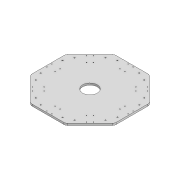
# Autodesk Inventor part: Base
Saved by Autodesk Inventor 2020 (Build 240168000, 168)
## iProperties
Created: 2022-03-01
Part Number: Base
Material: Generic
Document SubType Name: Modeling
Designer: ferrerx
Density: 1 g/cm^3
Appearance: Default
Author: ferrerx
Autodesk Inventor part; units mm, degrees
ref_plane "YZ Plane" through (0, 0, 0) normal (1, 0, 0) x (0, 1, 0)
ref_plane "XZ Plane" through (0, 0, 0) normal (0, 1, 0) x (-1, 0, 0)
ref_plane "XY Plane" through (0, 0, 0) normal (0, 0, 1) x (1, 0, 0)
sketch "Sketch1" plane through (0, 0, 0) normal (0, 1, 0) x (-1, 0, 0)
  circle A0 centre (0, 0) radius 20
  circle A1 centre (0, 0) radius 92.5 construction
  line L0 (115, -37.3658) -> (71.0739, -97.8248) construction
  line L1 (71.0739, -97.8248) -> (0, -120.9182) construction
  line L2 (0, -120.9182) -> (-71.0739, -97.8248) construction
  line L3 (-71.0739, -97.8248) -> (-115, -37.3658) construction
  line L4 (-115, -37.3658) -> (-115, 37.3658) construction
  line L5 (-115, 37.3658) -> (-71.0739, 97.8248) construction
  line L6 (-71.0739, 97.8248) -> (0, 120.9182) construction
  line L7 (0, 120.9182) -> (71.0739, 97.8248) construction
  line L8 (71.0739, 97.8248) -> (115, 37.3658) construction
  line L9 (115, 37.3658) -> (115, -37.3658) construction
  line L10 (0, 0) -> (0, -190.4975) construction
  line L11 (47.7367, -114.9577) -> (-47.5324, -115.0423)
  line L12 (-47.5324, -115.0423) -> (-114.9577, -47.7367)
  line L13 (-114.9577, -47.7367) -> (-115.0423, 47.5324)
  line L14 (-115.0423, 47.5324) -> (-47.7367, 114.9577)
  line L15 (-47.7367, 114.9577) -> (47.5324, 115.0423)
  line L16 (47.5324, 115.0423) -> (114.9577, 47.7367)
  line L17 (114.9577, 47.7367) -> (115.0423, -47.5324)
  line L18 (115.0423, -47.5324) -> (47.7367, -114.9577)
  dimension "d0" = 40
  dimension "d1" = 185
  dimension "d4" = 230
  dimension "d18" = 230
  constraints: 38 end point, 4 coincident, 2 centre point, 1 parallel, 1 vertical, 38 other
  measures "d0" diameter of A0
  measures "d1" diameter of A1
  measures "d4" distance between parallel lines of L4 L9
  measures "d18" distance between parallel lines of L15 L11
extrude "Extrusion1" add sketch "Sketch1" along normal blind 5
sketch "Sketch2" plane through (0, 5, 0) normal (0, 1, 0) x (1, 0, 0)
  line L0 (0, 0) -> (-100, 0) construction
  line L1 (-111.25, -6.75) -> (-88.75, -6.75) construction
  line L2 (-88.75, -6.75) -> (-88.75, 6.75) construction
  line L3 (-88.75, 6.75) -> (-111.25, 6.75) construction
  line L4 (-111.25, 6.75) -> (-111.25, -6.75) construction
  line L5 (-111.25, -6.75) -> (-88.75, 6.75) construction
  line L6 (-88.75, -6.75) -> (-111.25, 6.75) construction
  circle A0 centre (-111.25, -6.75) radius 1
  circle A1 centre (-111.25, 6.75) radius 1
  circle A2 centre (-88.75, 6.75) radius 1
  circle A3 centre (-88.75, -6.75) radius 1
  line L7 (-115, 37.3658) -> (-115, -37.3658) projected
  line L8 (-115.0423, 47.5324) -> (-114.9577, -47.7367) projected
  dimension "d5" = 22.5
  dimension "d6" = 13.5
  dimension "d7" = 2
  dimension "d8" = 2
  dimension "d9" = 2
  dimension "d10" = 2
  dimension "d19" = 15
  constraints: 14 end point, 4 centre point, 4 coincident, 2 horizontal, 2 midpoint, 2 parallel, 1 perpendicular
  measures "d5" distance of L2.end L3.end
  measures "d6" distance of L3.end L1.start
  measures "d7" diameter of A3
  measures "d8" diameter of A2
  measures "d9" diameter of A1
  measures "d10" diameter of A0
  measures "d19" distance from line of L0.end L8
extrude "Extrusion2" cut sketch "Sketch2" against normal blind 5
pattern_circular "Circular Pattern1" count 8 over 360 about axis through (0, 0, 0) along (0, 1, 0) of "Extrusion2"
fillet "Fillet1" radius 10 8 edges at (-47.5324, 2.5, 115.0423) (47.7367, 2.5, 114.9577) (115.0423, 2.5, 47.5324) (114.9577, 2.5, -47.7367) (47.5324, 2.5, -115.0423) (-47.7367, 2.5, -114.9577) (-115.0423, 2.5, -47.5324) (-114.9577, 2.5, 47.7367)
sketch "Sketch3" plane through (0, 5, 0) normal (0, 1, 0) x (1, 0, 0)
  circle A0 centre (-104.9734, -30) radius 1.5
  line L0 (-115.0386, 43.3903) -> (-114.9613, -43.5945) projected
  line L1 (0, 0) -> (-115, -0.1021)
  line L2 (0, 0) -> (-115, -0.1021)
  line L3 (-115, -0.1021) -> (-139, -0.1021) construction
  circle A1 centre (-104.9734, 29.7958) radius 1.5
  dimension "d22" = 3
  dimension "d23" = 30
  dimension "d24" = 10
  constraints: 6 end point, 2 centre point, 1 horizontal, 1 midpoint, 1 symmetric about line, 1 other
  measures "d22" diameter of A0
  measures "d23" vertical distance of L1.start A0.centre
  measures "d24" distance from line of L0 A0.centre
extrude "Extrusion3" cut sketch "Sketch3" against normal blind 10
pattern_circular "Circular Pattern2" count 8 over 360 about axis through (0, 0, 0) along (0, 1, 0) of "Extrusion3"
body "Solid1"
